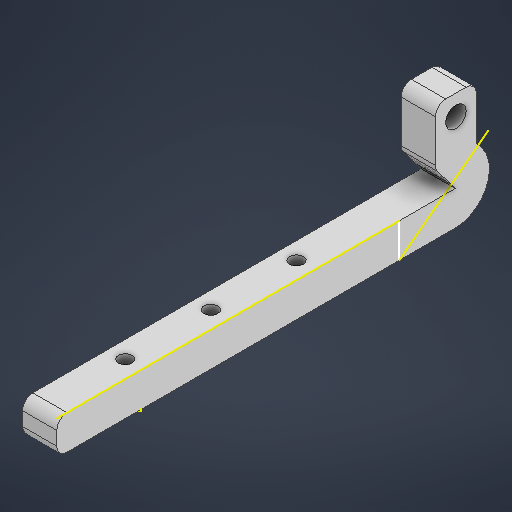
# Autodesk Inventor part: rod
Saved by Autodesk Inventor 2026.2 (Build 302298000, 298)
## iProperties
Created: 2025-12-16
Part Number: rod
Material: Generic
Document SubType Name: Modeling
Designer: Thoma
Density: 1 g/cm^3
Appearance: Default
Mass: 13.0768 g
Surface Area: 62.8747 cm^2
Volume: 13.0768 cm^3
Author: Thoma
Autodesk Inventor part; units mm, degrees
ref_plane "YZ Plane" through (0, 0, 0) normal (1, 0, 0) x (0, 1, 0)
ref_plane "XZ Plane" through (0, 0, 0) normal (0, 1, 0) x (-1, 0, 0)
ref_plane "XY Plane" through (0, 0, 0) normal (0, 0, 1) x (1, 0, 0)
sketch "Sketch1" plane through (0, 0, 0) normal (0, 1, 0) x (-1, 0, 0)
  line L0 (2.3256, 24.4186) -> (-7.6744, 24.4186)
  line L1 (-7.6744, 24.4186) -> (-7.6744, -75.5814)
  line L2 (-7.6744, -75.5814) -> (2.3256, -75.5814)
  line L3 (2.3256, -75.5814) -> (2.3256, 24.4186)
  point P0 (0, 0)
  dimension "d2" = 100
  dimension "d3" = 10
  constraints: 8 end point, 2 parallel, 1 horizontal, 1 perpendicular
  measures "d2" distance of L2.end L0.start
  measures "d3" distance of L0.start L0.end
extrude "Extrusion1" add sketch "Sketch1" along normal blind 10
sketch "Sketch9" plane through (7.6744, 0, 24.4186) normal (1, 0, 0) x (0, 0, -1)
  line L0 (0, 10) -> (100, 10) projected
  line L1 (0, 0) -> (100, 0) projected
  line L2 (0, 10) -> (100, 10)
  line L3 (100, 10) -> (100, 0)
  line L4 (100, 0) -> (0, 0)
  line L5 (0, 0) -> (0, 10)
  point P0 (24.4186, 0)
  constraints: 8 end point, 2 parallel, 1 horizontal, 1 perpendicular
extrude "Extrusion8" cut sketch "Sketch9" against normal blind 5
sketch "Sketch10" plane through (2.6744, 0, 24.4186) normal (1, 0, 0) x (0, 0, -1)
  line L0 (100, 0) -> (100, 10) projected
  line L1 (100, 10) -> (126, 10)
  line L2 (126, 10) -> (126, 29.842)
  line L3 (126, 29.842) -> (100, 10)
  line L4 (126, 29.842) -> (126, 19.842)
  line L5 (126, 19.842) -> (100, 0)
  point P0 (24.4186, 0)
  dimension "d44" = 19.842
  dimension "d45" = 26
  dimension "d46" = 10
  constraints: 10 end point, 1 horizontal, 1 perpendicular, 1 point on line
  measures "d44" distance of L1.end L2.end
  measures "d45" distance of L0.end L1.end
  measures "d46" distance of L2.end L4.end
extrude "Extrusion9" add sketch "Sketch10" against normal blind 5 contours L0 L1 L5 | L3 L2 L5 L1
sketch "Sketch12" plane through (2.6744, 0, 24.4186) normal (1, 0, 0) x (0, 0, -1)
  line L0 (100, 0) -> (0, 0) projected
  line L1 (126, 29.842) -> (126, 19.842) projected
  line L2 (99.9331, 0) -> (126, 19.842)
  line L3 (126, 19.842) -> (126, 29.842)
  line L4 (126, 29.842) -> (99.9331, 10)
  line L5 (99.9331, 10) -> (99.9331, 0)
  point P0 (24.4186, 0)
  constraints: 8 end point, 3 equal length
extrude "Extrusion10" add sketch "Sketch12" along normal blind 5
sketch "Sketch13" plane through (2.6744, 0, 24.4186) normal (1, 0, 0) x (0, 0, -1)
  line L0 (100, 10) -> (0, 10) projected
  line L1 (100, 0) -> (0, 0) projected
  line L2 (0, 10) -> (100, 10)
  line L3 (100, 10) -> (100, 0)
  line L4 (100, 0) -> (0, 0)
  line L5 (0, 0) -> (0, 10)
  point P0 (24.4186, 0)
  constraints: 8 end point, 2 parallel, 1 horizontal, 1 perpendicular
extrude "Extrusion11" add sketch "Sketch13" along normal blind 5
sketch "Sketch2" plane through (0, 10, 0) normal (0, 1, 0) x (1, 0, 0)
  line L0 (-2.3256, -24.4186) -> (7.6744, -24.4186) projected
  line L1 (7.6744, -24.4186) -> (7.6744, 75.5814) projected
  line L2 (-2.3256, -24.4186) -> (7.6744, -24.4186)
  line L3 (2.6744, -24.4186) -> (2.6744, -14.4186)
  line L4 (2.6744, -14.4186) -> (2.6744, -4.4186)
  line L5 (2.6744, -4.4186) -> (2.6744, 10.5814)
  line L6 (2.6744, 10.5814) -> (2.6744, 25.5814)
  line L7 (7.6744, 75.5814) -> (-2.3256, 75.5814) projected
  line L8 (-2.3256, 75.5814) -> (7.6744, 75.5814)
  line L9 (2.6744, -24.4186) -> (2.6744, 25.5814)
  line L10 (2.6744, 25.5814) -> (7.6744, 25.5814)
  line L11 (2.6744, 25.5814) -> (-2.3256, 25.5814)
  line L12 (-2.3256, 75.5814) -> (-2.3256, -24.4186) projected
  line L13 (2.6744, 25.5814) -> (2.6744, 40.5814)
  line L14 (2.6744, 25.5814) -> (2.6744, 75.5814)
  line L15 (2.6744, 0.5814) -> (-2.3256, 0.5814)
  line L16 (2.6744, 0.5814) -> (7.6744, 0.5814)
  line L17 (2.6744, 50.5814) -> (-2.3256, 50.5814)
  line L18 (7.6744, 50.5814) -> (2.6744, 50.5814)
  circle A0 centre (2.6744, 0.5814) radius 2
  circle A1 centre (2.6744, 25.5814) radius 2
  circle A2 centre (2.6744, 50.5814) radius 2
  point P0 (0, 0)
  dimension "d28" = 4
  dimension "d29" = 4
  dimension "d30" = 4
  constraints: 30 end point, 6 midpoint, 6 point on line, 5 coincident, 5 vertical, 3 centre point, 2 collinear, 2 perpendicular, 1 horizontal
  measures "d28" diameter of A0
  measures "d29" diameter of A1
  measures "d30" diameter of A2
extrude "Extrusion2" cut sketch "Sketch2" against normal blind 10 contours A0 L5 L15 | L15 L5 A0 | A1 L13 L11 | L11 L6 A1 | L16 A0 L5 | L5 A0 L16 | L10 A1 L6 | L13 A1 L10 | A2 L14 L17 | L17 L14 A2 | L18 A2 L14 | L14 A2 L18
sketch "Sketch14" plane through (7.6744, 0, 24.4186) normal (1, 0, 0) x (0, 0, -1)
  line L0 (100, 10) -> (0, 10) projected
  line L1 (126, 19.842) -> (100, 0) projected
  line L2 (100, 10) -> (100, 0)
  point P0 (24.4186, 0)
  constraints: 2 end point, 1 vertical
sketch "Sketch16" plane through (7.6744, 0, 24.4186) normal (1, 0, 0) x (0, 0, -1)
  line L0 (100, 10) -> (126, 29.842) projected
  line L1 (100, 10) -> (112.8965, 19.842)
  line L2 (112.8965, 19.842) -> (113.5142, 20.3134)
  line L3 (113.5142, 20.3134) -> (118.3291, 14.0042)
  line L4 (117.7114, 13.5328) -> (112.8841, 19.8582) projected
  line L5 (117.7114, 13.5328) -> (118.3291, 14.0042)
  point P0 (24.4186, 0)
  dimension "d60" = 16.223
  dimension "d61" = 0.7771
  constraints: 8 end point, 1 collinear, 1 parallel, 1 point on line
  measures "d60" distance of L0.start L1.end
  measures "d61" distance of L1.end L2.end
extrude "Extrusion13" add sketch "Sketch16" against normal blind 10
sketch "Sketch20" plane through (7.6744, 0, 24.4186) normal (1, 0, 0) x (0, 0, -1)
  line L0 (100, 10) -> (0, 10) projected
  line L1 (100, 10) -> (128, 10)
  line L2 (128, 10) -> (128, 0)
  line L3 (128, 0) -> (100, 0)
  line L4 (100, 0) -> (100, 10)
  line L5 (126, 29.842) -> (100, 10) projected
  line L6 (100, 10) -> (126, 10)
  line L7 (126, 10) -> (126, 29.842)
  line L8 (126, 29.842) -> (100, 29.842)
  line L9 (100, 29.842) -> (100, 10)
  point P0 (24.4186, 0)
  dimension "d77" = 28
  constraints: 16 end point, 4 parallel, 2 horizontal, 2 perpendicular
  measures "d77" distance of L2.end L3.end
extrude "Extrusion17" add sketch "Sketch20" against normal blind 10 contours L1 L2 L3 L4
sketch "Sketch21" plane through (7.6744, 0, 24.4186) normal (1, 0, 0) x (0, 0, -1)
  line L0 (128, 0) -> (128, 10) projected
  line L1 (128, 0) -> (151.8705, 18.1701)
  line L2 (113.0703, 10) -> (126, 19.842) projected
  line L3 (128, 10) -> (151.2395, 27.6897)
  line L4 (151.8705, 18.1701) -> (151.8705, 28.1701)
  line L5 (151.8705, 28.1701) -> (151.2395, 27.6897)
  line L6 (100, 10) -> (0, 10) projected
  line L7 (126, 29.842) -> (100, 29.842)
  line L8 (100, 29.842) -> (100, 10)
  line L9 (100, 10) -> (126, 10)
  line L10 (126, 10) -> (126, 29.842)
  point P0 (24.4186, 0)
  constraints: 16 end point, 4 parallel, 1 collinear, 1 horizontal, 1 perpendicular, 1 vertical
extrude "Extrusion18" add sketch "Sketch21" against normal blind 10 contours L0 L3 L5 L4 L1
sketch "Sketch22" plane through (7.6744, 0, 24.4186) normal (1, 0, 0) x (0, 0, -1)
  line L0 (100, 10) -> (126, 29.842) projected
  line L1 (100, 10) -> (0, 10) projected
  line L2 (126, 29.842) -> (100, 29.842)
  line L3 (100, 29.842) -> (100, 10)
  line L4 (100, 10) -> (126, 10)
  line L5 (126, 10) -> (126, 29.842)
  point P0 (24.4186, 0)
  constraints: 8 end point, 2 parallel, 1 horizontal, 1 perpendicular
extrude "Extrusion19" cut sketch "Sketch22" against normal blind 10
sketch "Sketch23" plane through (7.6744, 0, 24.4186) normal (1, 0, 0) x (0, 0, -1)
  line L0 (151.8705, 18.1701) -> (128, 0) projected
  line L1 (141.8914, 10.574) -> (136.9966, 17.0044)
  line L2 (128, 0) -> (151.8705, 18.1701) projected
  line L3 (128, 10) -> (151.8705, 28.1701) projected
  line L4 (137.0719, 16.9055) -> (151.8705, 28.1701)
  line L5 (151.8705, 28.1701) -> (151.8705, 18.1701)
  line L6 (141.8914, 10.574) -> (151.8705, 18.1701)
  point P0 (24.4186, 0)
  point P1 (137.0719, 16.9055)
  constraints: 8 end point, 2 collinear, 2 point on line, 1 perpendicular, 1 vertical
extrude "Extrusion20" cut sketch "Sketch23" against normal blind 10
sketch "Sketch24" plane through (7.6744, 0, 24.4186) normal (1, 0, 0) x (0, 0, -1)
  line L0 (141.8914, 10.574) -> (137.0719, 16.9055) projected
  line L1 (137.0719, 16.9055) -> (120.0422, 39.2779)
  line L2 (120.0422, 39.2779) -> (114.7811, 35.2732)
  line L3 (114.7811, 35.2732) -> (131.8109, 12.9008)
  line L4 (128, 10) -> (137.0719, 16.9055) projected
  line L5 (130.4337, 25.6264) -> (125.1726, 21.6217)
  point P0 (24.4186, 0)
  constraints: 8 end point, 3 perpendicular, 3 point on line, 1 collinear
extrude "Extrusion21" add sketch "Sketch24" against normal blind 10 contours L4 L3 L5 L1
sketch "Sketch25" plane through (7.6744, 0, 24.4186) normal (1, 0, 0) x (0, 0, -1)
  circle A0 centre (130.0281, 20.9631) radius 1.4142
  line L0 (128, 0) -> (141.8914, 10.574) projected
  point P0 (24.4186, 0)
  dimension "d88" = 15.452
  constraints: 1 centre point
  measures "d88" distance from line of L0 A0.centre
extrude "Extrusion22" cut sketch "Sketch25" against normal blind 10
sketch "Sketch26" plane through (7.6744, 0, 24.4186) normal (1, 0, 0) x (0, 0, -1)
  line L0 (146.1805, 13.3852) -> (129.0054, 0.3116)
  line L1 (128, 0) -> (141.8914, 10.574) projected
  line L2 (129.0054, 0.3116) -> (127.1011, -1.1379)
  line L3 (128, 0) -> (128.596, 0)
  line L4 (128, 10) -> (141.7333, 10)
  point P0 (24.4186, 0)
  point P1 (137.593, 6.8484)
  point P2 (141.1373, 10)
  dimension "d89" = 0.361
  constraints: 8 end point, 2 parallel, 2 point on line, 1 collinear, 1 horizontal, 1 midpoint
  measures "d89" distance from line of point (137.593, 6.848) L1
extrude "Extrusion23" add sketch "Sketch26" against normal blind 10
sketch "Sketch27" plane through (7.6744, 0, 24.4186) normal (1, 0, 0) x (0, 0, -1)
  line L0 (128.596, 0) -> (141.7333, 10) projected
  line L1 (141.7333, 10) -> (143.6446, 11.4549)
  line L2 (141.7333, 10) -> (141.1373, 10) projected
  line L3 (141.7333, 10) -> (141.1373, 10)
  line L4 (141.1373, 10) -> (143.4259, 11.7421)
  line L5 (143.4259, 11.7421) -> (143.6446, 11.4549)
  line L6 (143.4259, 11.7421) -> (141.6084, 14.1298)
  line L7 (141.6084, 14.1298) -> (140.0739, 12.9618)
  line L8 (130.4337, 25.6264) -> (141.8914, 10.574) projected
  line L9 (141.8914, 10.574) -> (140.0739, 12.9618)
  line L10 (141.8914, 10.574) -> (130.4337, 25.6264) projected
  point P0 (24.4186, 0)
  dimension "d92" = 2.402
  constraints: 14 end point, 4 perpendicular, 3 point on line, 2 collinear, 1 parallel
  measures "d92" distance of L0.end L1.end
extrude "Extrusion24" add sketch "Sketch27" against normal blind 10
sketch "Sketch28" plane through (7.6744, 0, 24.4186) normal (1, 0, 0) x (0, 0, -1)
  line L0 (129.7749, 26.8286) -> (140.6808, 12.5013)
  line L1 (140.0739, 12.9618) -> (130.4337, 25.6264) projected
  line L2 (130.4337, 25.6264) -> (130.596, 25.7499)
  line L3 (140.0739, 12.9618) -> (141.6084, 14.1298) projected
  line L4 (140.0739, 12.9618) -> (140.2362, 13.0853)
  line L5 (140.0739, 12.9618) -> (130.4337, 25.6264)
  point P0 (24.4186, 0)
  dimension "d95" = 0.204
  constraints: 8 end point, 3 point on line, 1 collinear, 1 parallel, 1 perpendicular
  measures "d95" distance between parallel lines of L0 L1
extrude "Extrusion25" add sketch "Sketch28" against normal blind 10
sketch "Sketch29" plane through (7.6744, 0, 24.4186) normal (1, 0, 0) x (0, 0, -1)
  line L0 (130.596, 25.7499) -> (140.2362, 13.0853) projected
  line L1 (130.596, 25.7499) -> (115.0002, 13.8785)
  line L2 (143.6446, 11.4549) -> (128.596, 0) projected
  line L3 (137.4941, 6.7732) -> (119.5658, 30.326)
  line L4 (122.7981, 19.8142) -> (116.5462, 28.0275)
  circle A0 centre (116.5462, 28.0275) radius 3
  line L5 (116.5462, 28.0275) -> (116.5462, 10)
  line L6 (0, 10) -> (128, 10) projected
  line L7 (128, 10) -> (100, 10) projected
  line L8 (116.5462, 28.0275) -> (110.5462, 28.0275)
  line L9 (110.5462, 28.0275) -> (110.5462, 34.0275)
  line L10 (116.5462, 28.0275) -> (122.5462, 28.0275)
  line L11 (122.5462, 28.0275) -> (122.5462, 10)
  line L12 (110.5462, 34.0275) -> (122.5462, 34.0275)
  line L13 (122.5462, 34.0275) -> (122.5462, 10)
  line L14 (122.5462, 10) -> (110.5462, 10)
  line L15 (110.5462, 10) -> (110.5462, 34.0275)
  point P0 (24.4186, 0)
  point P1 (122.5462, 28.0275)
  point P2 (110.5462, 28.0275)
  point P3 (110.5462, 10)
  point P4 (122.5462, 10)
  dimension "d98" = 19.6
  dimension "d99" = 29.6
  dimension "d100" = 6
  dimension "d101" = 6
  dimension "d102" = 6
  dimension "d103" = 6
  constraints: 24 end point, 5 perpendicular, 3 horizontal, 3 parallel, 3 point on line, 2 vertical, 1 centre point, 1 coincident, 1 midpoint
  measures "d98" distance of L0.start L1.end
  measures "d99" distance of L3.start L3.end
  measures "d100" diameter of A0
  measures "d101" distance of L5.start L8.end
  measures "d102" distance of L8.end L9.end
  measures "d103" distance of L5.start L10.end
extrude "Extrusion26" add sketch "Sketch29" against normal blind 10 contours L11 L4 A0 L10 L3 | L3 L10 L11 | L11 L6 L5 L1 | L1 L5 A0 L4 L11 | L10 A0 L8 L9 L12 L13 | L5 L6 L15 L8 A0
sketch "Sketch30" plane through (7.6744, 0, 24.4186) normal (1, 0, 0) x (0, 0, -1)
  line L0 (122.5462, 34.0275) -> (122.5462, 10) projected
  line L1 (122.5462, 34.0275) -> (144, 34.0275)
  line L2 (144, 34.0275) -> (144, 0)
  line L3 (144, 0) -> (122.5462, 0)
  line L4 (122.5462, 0) -> (122.5462, 34.0275)
  point P0 (24.4186, 0)
  constraints: 8 end point, 2 parallel, 1 horizontal, 1 perpendicular
extrude "Extrusion27" cut sketch "Sketch30" against normal blind 10
sketch "Sketch31" plane through (7.6744, 0, 24.4186) normal (1, 0, 0) x (0, 0, -1)
  line L0 (110.5462, 34.0275) -> (110.5462, 10) projected
  line L1 (110.5462, 10) -> (113, 10)
  line L2 (110.5462, 10) -> (114, 10)
  line L3 (114, 10) -> (114, 17)
  line L4 (114, 17) -> (110.5462, 17)
  line L5 (110.5462, 17) -> (110.5462, 10)
  point P0 (24.4186, 0)
  constraints: 10 end point, 2 horizontal, 2 parallel, 1 perpendicular
extrude "Extrusion28" cut sketch "Sketch31" against normal blind 10
sketch "Sketch32" plane through (7.6744, 0, 24.4186) normal (1, 0, 0) x (0, 0, -1)
  line L0 (114, 17) -> (110.5462, 17) projected
  line L1 (114, 17) -> (114, 10) projected
  line L2 (110.5462, 17) -> (114, 10)
  line L3 (114, 10) -> (114, 17)
  line L4 (114, 17) -> (110.5462, 17)
  point P0 (24.4186, 0)
  constraints: 6 end point, 1 collinear, 1 perpendicular
extrude "Extrusion29" add sketch "Sketch32" against normal blind 10
sketch "Sketch33" plane through (7.6744, 0, 24.4186) normal (1, 0, 0) x (0, 0, -1)
  line L0 (100, 10.051) -> (99.9331, 10) projected
  line L1 (100, 10.051) -> (99.9331, 10)
  line L2 (99.9331, 10) -> (100, 10) projected
  line L3 (99.9331, 10) -> (100, 10)
  line L4 (100, 10) -> (100, 10.051) projected
  line L5 (100, 10) -> (100, 10.051)
  point P0 (24.4186, 0)
  constraints: 6 end point, 2 collinear, 1 perpendicular
extrude "Extrusion30" cut sketch "Sketch33" against normal blind 10
sketch "Sketch34" plane through (7.6744, 0, 24.4186) normal (1, 0, 0) x (0, 0, -1)
  line L0 (119.6145, 21.221) -> (127.7254, 4.7823)
  line L1 (110.5462, 17) -> (114, 10) projected
  line L2 (127.7254, 4.7823) -> (130.085, 0)
  line L3 (122.5462, 0) -> (0, 0) projected
  line L4 (116.5047, 0) -> (130.085, 0)
  line L5 (127.7254, 4.7823) -> (130.085, 0)
  line L6 (122.5462, 34.0275) -> (122.5462, 0) projected
  line L7 (122.5462, 15.2793) -> (122.5462, 0)
  point P0 (24.4186, 0)
  dimension "d114" = 10
  constraints: 10 end point, 3 point on line, 2 collinear, 1 parallel, 1 perpendicular
  measures "d114" distance between parallel lines of L0 L1
extrude "Extrusion31" add sketch "Sketch34" against normal blind 10
fillet "Fillet2" radius 2 1 edges at (2.6744, 0, -105.6664)
fillet "Fillet3" radius 3 6 edges at (2.6744, 15.2793, -98.1276) (2.6744, 34.0275, -98.1276) (2.6744, 34.0275, -86.1276) (2.6744, 17, -86.1276) (2.6744, 10, 24.4186) (2.6744, 0, 24.4186)
sketch "Sketch35" plane through (7.6744, 0, 24.4186) normal (1, 0, 0) x (0, 0, -1)
  arc A0 (110.5462, 17.6998) -> (110.8558, 16.3724) centre (113.5462, 17.6998) ccw projected
  line L0 (110.5462, 17.6998) -> (115.9997, 10.0548)
  line L1 (115.9997, 10.0548) -> (113.9997, 10.0548)
  line L2 (110.5462, 17.6998) -> (110.5462, 10.0548)
  line L3 (110.5462, 10.0548) -> (115.9997, 10.0548)
  line L4 (114, 10) -> (3, 10) projected
  line L5 (110.5462, 10.0548) -> (115.9997, 10.0548)
  point P0 (24.4186, 0)
  point P1 (3, 10)
  constraints: 10 end point, 1 collinear, 1 horizontal, 1 perpendicular, 1 vertical, 1 other
extrude "Extrusion32" cut sketch "Sketch35" against normal blind 10
sketch "Sketch36" plane through (7.6744, 0, 24.4186) normal (1, 0, 0) x (0, 0, -1)
  line L0 (107, 10) -> (116.6574, 10)
  line L1 (110.5462, 17.6998) -> (115.9997, 10.0548) projected
  line L2 (3, 0) -> (126.868, 0) projected
  line L3 (126, 19.8421) -> (100, 0)
  line L4 (114.4821, 12.6317) -> (116.576, 9.6964)
  line L5 (115.2117, 11.6089) -> (109.4902, 19.1061)
  line L6 (110.5462, 31.0275) -> (110.5462, 17.6998) projected
  line L7 (110.5462, 17.6998) -> (110.5462, 10)
  line L8 (110.5462, 10) -> (116.3594, 10)
  point P0 (24.4186, 0)
  point P1 (110.5462, 17.7223)
  dimension "d121" = 0.261
  constraints: 12 end point, 6 point on line, 2 perpendicular, 1 horizontal, 1 parallel
  measures "d121" distance between parallel lines of L4 L1
extrude "Extrusion33" cut sketch "Sketch36" against normal blind 10
fillet "Fillet5" radius 3 1 edges at (2.6744, 17.7223, -86.1276)
sketch "Sketch37" plane through (7.6744, 0, 24.4186) normal (1, 0, 0) x (0, 0, -1)
  line L0 (117.9323, 24.5273) -> (136.6505, 0)
  line L1 (111.1613, 16.9163) -> (115.2117, 11.6089) projected
  line L2 (126.868, 0) -> (3, 0) projected
  line L3 (122.3182, 0) -> (151, 0)
  line L4 (122.5644, 18.4576) -> (122.5644, 0)
  line L5 (122, 19.1972) -> (122, 0)
  point P0 (24.4186, 0)
  dimension "d126" = 10
  constraints: 8 end point, 6 point on line, 2 perpendicular, 1 collinear, 1 parallel
  measures "d126" distance between parallel lines of L0 L1
extrude "Extrusion34" add sketch "Sketch37" against normal blind 10
fillet "Fillet6" radius 3 2 edges at (2.6744, 0, -112.2319) (2.6744, 18.4815, -98.1276)
sketch "Sketch38" plane through (7.6744, 0, 24.4186) normal (1, 0, 0) x (0, 0, -1)
  line L0 (116.3594, 10) -> (115.2117, 11.6089) projected
  circle A0 centre (116.3594, 10) radius 10
  line L1 (116.3594, 0) -> (138.2555, 0)
  line L2 (123.1613, 17.6755) -> (132.9721, 4.82) projected
  line L3 (125.5984, 14.4821) -> (136.6505, 0)
  line L4 (122.5462, 31.0275) -> (122.5462, 19.4955) projected
  line L5 (122.5462, 23.6272) -> (122.5462, 15.6271)
  line L6 (127.4926, 12) -> (119.861, 22)
  line L7 (122.5462, 18.3765) -> (125.8778, 14.0109)
  line L8 (132.9721, 4.82) -> (123.1613, 17.6755) projected
  line L9 (122.5462, 18.3765) -> (122.5462, 19.4955)
  line L10 (136.6505, 0) -> (122.5462, 19.4955)
  point P0 (24.4186, 0)
  point P1 (124.3089, 16.0667)
  dimension "d130" = 20
  constraints: 14 end point, 6 point on line, 3 collinear, 2 horizontal, 2 parallel, 4 other
extrude "Extrusion35" cut sketch "Sketch38" against normal blind 10 contours A0 L7 L5 L6 L2 L3 L1 | L3 L2 L6 L5 L10
sketch "Sketch39" plane through (7.6744, 0, 24.4186) normal (1, 0, 0) x (0, 0, -1)
  point P0 (24.4186, 0)
equation "\"d0\" = d3"
body "Solid1"
